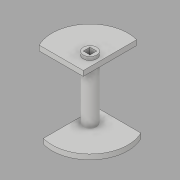
# Autodesk Inventor part: DispenserAugerV2
Saved by Autodesk Inventor 2017 (Build 210142000, 142)
## iProperties
Created: 2017-02-22
Part Number: DispenserAugerV2
Material: Generic
Document SubType Name: Modeling
Designer: gmarsh
Density: 1 g/cm^3
Appearance: Default
Author: gmarsh
Autodesk Inventor part; units mm, degrees
ref_plane "YZ Plane" through (0, 0, 0) normal (1, 0, 0) x (0, 1, 0)
ref_plane "XZ Plane" through (0, 0, 0) normal (0, 1, 0) x (-1, 0, 0)
sketch "Sketch1" plane through (0, 0, 0) normal (0, 0, 1) x (1, 0, 0)
  circle A0 centre (0, 0) radius 4
  constraints: 1 centre point
extrude "Extrusion1" add sketch "Sketch1" along normal blind 40
ref_plane "Work Plane5" through (0, 0, 35) normal (0, 0, 1) x (1, 0, 0)
sketch "Sketch5" plane through (0, 0, 35) normal (0, 0, 1) x (1, 0, 0)
  arc A0 (6, 21.6852) -> (-20.1556, -10) centre (0, 0) ccw
  line L0 (-20.1556, -10) -> (6, -10)
  line L1 (6, 21.6852) -> (6, -10)
  dimension "d19" = 45
  constraints: 4 end point, 2 point on circle, 1 centre point, 1 horizontal, 1 perpendicular
  measures "d19" diameter of A0
extrude "Extrusion4" add sketch "Sketch5" along normal blind 3
sketch "Sketch6" plane through (0, 0, 0) normal (0, 0, -1) x (-1, 0, 0)
  arc A0 (-20.1556, 10) -> (6, -21.6852) centre (0, 0) ccw
  line L0 (6, 10) -> (-20.1556, 10)
  line L1 (6, 10) -> (6, -21.6852)
  dimension "d20" = 45
  constraints: 4 end point, 2 point on circle, 1 centre point, 1 horizontal, 1 vertical
  measures "d20" diameter of A0
extrude "Extrusion5" add sketch "Sketch6" against normal blind 3 separate body
sketch "Sketch3" plane through (0, 0, 0) normal (0, 0, -1) x (-1, 0, 0)
  line L0 (2, 2) -> (-2, 2)
  line L1 (-2, 2) -> (-2, -2)
  line L2 (-2, -2) -> (2, -2)
  line L3 (2, -2) -> (2, 2)
  line L4 (2, 2) -> (-2, -2) construction
  line L5 (-2, 2) -> (2, -2) construction
  point P0 (0, 0)
  dimension "d5" = 4
  dimension "d6" = 4
  constraints: 12 end point, 2 midpoint, 2 parallel, 1 horizontal, 1 perpendicular
  measures "d5" distance of L2.end L1.end
  measures "d6" distance of L1.end L0.end
extrude "Extrusion3" cut sketch "Sketch3" against normal blind 40 and the other way blind 5 bodies 1 2
body "Solid1"
body "Solid2"
